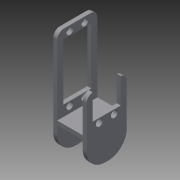
# Autodesk Inventor part: new_leg_2
Saved by Autodesk Inventor 2014 SP1 (Build 180222100, 222)
## iProperties
Created: 2014-12-05
Part Number: new_leg_2
Material: Générique
Document SubType Name: Modeling
Designer: astralien3000
Density: 1 g/cm^3
Appearance: Par défaut
d0: 3,000 mm
d1: 3,000 mm
d2: 3,000 mm
d4: 25,000 mm
d5: 80,000 mm
d6: 40,000 mm
d7: 12,500 mm
d11: 57,000 mm
d12: 30,000 mm
d13: 30,000 mm
d14: 0,00 deg
d15: 14,000 mm
d16: 21,000 mm
d17: 10,500 mm
d18: 7,000 mm
d19: 42,000 mm
d21: 7,000 mm
d22: 5,000 mm
d23: 4,900 mm
d24: 3,800 mm
d25: 5,000 mm
d26: 5,000 mm
d27: 5,000 mm
d28: 3,800 mm
d29: 4,900 mm
d30: 3,800 mm
d31: 4,900 mm
d32: 3,800 mm
d33: 4,900 mm
d35: 0,00 deg
d36: 5,000 mm
d37: 5,000 mm
d38: 5,000 mm
d39: 5,000 mm
d20: 7,000 mm
Author: astralien3000
Autodesk Inventor part; units mm, degrees
ref_plane "YZ Plane" through (0, 0, 0) normal (1, 0, 0) x (0, 1, 0)
ref_plane "XZ Plane" through (0, 0, 0) normal (0, 1, 0) x (-1, 0, 0)
ref_plane "XY Plane" through (0, 0, 0) normal (0, 0, 1) x (1, 0, 0)
sketch "Esquisse1" plane through (0, 0, 0) normal (0, 1, 0) x (-1, 0, 0)
  line L0 (-9.5, -40) -> (-12.5, -40)
  line L1 (-12.5, -40) -> (-12.5, 10)
  line L2 (-12.5, 10) -> (-9.5, 10)
  line L3 (-9.5, 10) -> (-9.5, -40)
  line L4 (9.5, 40) -> (12.5, 40)
  line L5 (12.5, 40) -> (12.5, -40)
  line L6 (12.5, -40) -> (9.5, -40)
  line L7 (9.5, -40) -> (9.5, 40)
  line L8 (-9.5, -20) -> (9.5, -20)
  line L9 (9.5, -20) -> (9.5, -17)
  line L10 (9.5, -17) -> (-9.5, -17)
  line L11 (-9.5, -17) -> (-9.5, -20)
  point P0 (0, 0)
  dimension "d0" = 3
  dimension "d1" = 3
  dimension "d2" = 3
  dimension "d4" = 25
  dimension "d5" = 80
  dimension "d6" = 40
  dimension "d7" = 12.5
  dimension "d11" = 57
  dimension "d12" = 30
  constraints: 24 end point, 6 parallel, 3 horizontal, 3 perpendicular, 2 point on line, 1 collinear
  measures "d0" distance between parallel lines of L7 L5
  measures "d1" distance between parallel lines of L1 L3
  measures "d2" distance between parallel lines of L8 L10
  measures "d4" distance between parallel lines of L5 L1
  measures "d5" distance between parallel lines of L6 L4
  measures "d6" vertical distance of point (0, 0) L5.end
  measures "d7" distance from line of point (0, 0) L5
  measures "d11" distance between parallel lines of L10 L4
  measures "d12" distance between parallel lines of L4 L2
extrude "Extrusion1" add sketch "Esquisse1" along normal blind 30
fillet "Congé1" radius 14 4 edges at (11, 30, -40) (-11, 30, -40) (11, 0, -40) (-11, 0, -40)
sketch "Esquisse2" plane through (-12.5, 0, 40) normal (-1, 0, 0) x (0, 0, 1)
  line L0 (0, 0) -> (0, 30) projected
  line L1 (-80, 14) -> (-80, 16) projected
  line L2 (-49, 25.5) -> (-7, 25.5)
  line L3 (-7, 25.5) -> (-7, 4.5)
  line L4 (-7, 4.5) -> (-49, 4.5)
  line L5 (-49, 4.5) -> (-49, 25.5)
  line L6 (0, 15) -> (-80, 15) construction
  line L7 (-7, 25.5) -> (0, 25.5) construction
  line L8 (0, 25.5) -> (0, 4.5) construction
  line L9 (0, 4.5) -> (-7, 4.5) construction
  line L10 (-7, 4.5) -> (-7, 25.5) construction
  line L11 (-49, 25.5) -> (-56, 25.5) construction
  line L12 (-56, 25.5) -> (-56, 4.5) construction
  line L13 (-56, 4.5) -> (-49, 4.5) construction
  line L14 (-49, 4.5) -> (-49, 25.5) construction
  circle A0 centre (-52.2, 20.6) radius 2.5
  circle A1 centre (-52.2, 9.4) radius 2.5
  circle A2 centre (-3.8, 9.4) radius 2.5
  circle A3 centre (-3.8, 20.6) radius 2.5
  point P0 (-40, 0)
  dimension "d16" = 21
  dimension "d17" = 10.5
  dimension "d18" = 7
  dimension "d19" = 42
  dimension "d20" = 7
  dimension "d21" = 7
  dimension "d22" = 5
  dimension "d23" = 4.9
  dimension "d24" = 3.8
  dimension "d25" = 5
  dimension "d26" = 5
  dimension "d27" = 5
  dimension "d28" = 3.8
  dimension "d29" = 4.9
  dimension "d30" = 3.8
  dimension "d31" = 4.9
  dimension "d32" = 3.8
  dimension "d33" = 4.9
  constraints: 26 end point, 6 parallel, 4 centre point, 3 horizontal, 3 perpendicular, 2 collinear, 2 midpoint, 1 point on line
  measures "d16" distance between parallel lines of L4 L2
  measures "d17" distance between parallel lines of L6 L4
  measures "d18" distance between parallel lines of L0 L3
  measures "d19" distance between parallel lines of L3 L5
  measures "d20" distance between parallel lines of L10 L8
  measures "d21" distance between parallel lines of L12 L5
  measures "d22" diameter of A0
  measures "d23" distance from line of L11 A0.centre
  measures "d24" distance from line of L12 A0.centre
  measures "d25" diameter of A1
  measures "d26" diameter of A2
  measures "d27" diameter of A3
  measures "d28" distance from line of L12 A1.centre
  measures "d29" distance from line of L13 A1.centre
  measures "d30" distance from line of L0 A2.centre
  measures "d31" distance from line of L9 A2.centre
  measures "d32" distance from line of L0 A3.centre
  measures "d33" distance from line of L7 A3.centre
extrude "Extrusion2" cut sketch "Esquisse2" against normal through all
fillet "Congé2" radius 5 1 edges at (-11, 0, 40)
fillet "Congé3" radius 5 1 edges at (-11, 30, 40)
fillet "Congé4" radius 5 1 edges at (11, 0, 10)
fillet "Congé5" radius 5 1 edges at (11, 30, 10)
equation "\"d6\" = 0.5 * d5"
equation "\"d7\" = 0.5 * d4"
equation "\"d17\" = 0.5 * d16"
equation "\"d21\" = d20"
equation "\"d25\" = d22"
equation "\"d26\" = d22"
equation "\"d27\" = d22"
equation "\"d28\" = d24"
equation "\"d29\" = d23"
equation "\"d30\" = d24"
equation "\"d31\" = d23"
equation "\"d32\" = d24"
equation "\"d33\" = d23"
